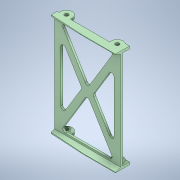
# Autodesk Inventor part: BodyStructure Plate
Saved by Autodesk Inventor 2022.2 (Build 262287000, 287)
## iProperties
Created: 2019-11-07
Part Number: BodyStructure Plate
Material: solidworks materials|ABS
Document SubType Name: Modeling
Designer: Jochen
Density: 1.02 g/cm^3
Appearance: 151,157,178
Sending System: SolidWorks 2017
Last Author: Felix
Last Saved: 2021-02-23
Author: Jochen
Autodesk Inventor part; units mm, degrees
ref_plane "YZ Plane" through (0, 0, 0) normal (1, 0, 0) x (0, 1, 0)
ref_plane "XZ Plane" through (0, 0, 0) normal (0, 1, 0) x (-1, 0, 0)
ref_plane "Work Plane1" through (0, 0, 30) normal (0, 0, 1) x (1, 0, 0)
sketch "Sketch1" plane through (0, 0, 30) normal (0, 0, 1) x (1, 0, 0)
  line L0 (-26, -40.5) -> (26, -40.5)
  line L1 (26, 40.5) -> (-26, 40.5)
  line L2 (26, 37) -> (26, 37)
  line L3 (0, -56.7) -> (0, 56.7) construction
  line L4 (-36.4, 0) -> (36.4, 0) construction
  line L5 (0, -2.5) -> (-21, -37)
  line L6 (-21, -27.3836) -> (-4.3317, 0)
  line L7 (-21, 27.3836) -> (-4.3317, 0)
  line L8 (0, 2.5) -> (-21, 37)
  line L9 (-26, 37) -> (-26, 37)
  line L10 (-21, 37) -> (21, 37)
  line L11 (-26, -37) -> (-26, -37)
  line L12 (21, -37) -> (-21, -37)
  line L13 (26, -37) -> (26, -37)
  line L14 (26, -40.5) -> (26, -37)
  line L15 (26, 37) -> (26, 40.5)
  line L16 (-26, 40.5) -> (-26, 37)
  line L17 (-26, -37) -> (-26, -40.5)
  line L18 (-26, -37) -> (-26, 37)
  line L19 (-21, -27.3836) -> (-21, 27.3836)
  line L20 (26, -37) -> (26, 37)
  line L21 (21, -27.3836) -> (21, 27.3836)
  line L22 (0, -2.5) -> (21, -37)
  line L23 (21, -27.3836) -> (4.3317, 0)
  line L24 (4.3317, 0) -> (21, 27.3836)
  line L25 (21, 37) -> (0, 2.5)
  point P0 (0, 0)
  point P1 (-5.9128, 0)
  dimension "d1" = 5
  dimension "d3" = 0
  dimension "d4" = 52
  dimension "d7" = 81
  dimension "d81" = 3.5
  dimension "d82" = 5
  dimension "d83" = 5
  dimension "d84" = 5
  constraints: 48 end point, 7 parallel, 6 horizontal, 5 collinear, 4 perpendicular, 4 point on line, 3 vertical, 1 coincident, 13 other
  measures "d1" distance between parallel lines of L6 L5
  measures "d3" distance of L11.start L11.end
  measures "d4" distance of L0.start L0.end
  measures "d7" distance between parallel lines of L1 L0
  measures "d81" distance of L11.end L0.start
  measures "d82" distance between parallel lines of L19 L18
  measures "d83" distance of L8.start L5.start
  measures "d84" distance of L5.end L11.start
extrude "Extrusion1" add sketch "Sketch1" along normal blind 13
fillet "Fillet1" radius 2 12 edges at (21, -37, 36.5) (0, -2.5, 36.5) (-21, -37, 36.5) (-4.3317, 0, 36.5) (-21, 37, 36.5) (21, 37, 36.5) (4.3317, 0, 36.5) (0, 2.5, 36.5) (21, -27.3836, 36.5) (-21, -27.3836, 36.5) (-21, 27.3836, 36.5) (21, 27.3836, 36.5)
sketch "Sketch3" plane through (0, 0, 0) normal (1, 0, 0) x (0, 1, 0)
  line L0 (0, -8.6) -> (0, 51.6) construction
  line L1 (-56.794, 0) -> (56.7157, 0) construction
  line L2 (-40.5, 43) -> (40.5, 43) construction
  line L3 (40.5, 43) -> (-40.5, 43) construction
  line L4 (21.2913, 43) -> (1.0399, 43) construction
  line L5 (-1.0399, 43) -> (1.0399, 43) construction
  line L6 (-1.0399, 43) -> (-21.2913, 43) construction
  line L7 (-1.0399, 30) -> (-21.2913, 30) construction
  line L8 (1.0399, 30) -> (-1.0399, 30) construction
  line L9 (21.2913, 30) -> (1.0399, 30) construction
  line L10 (40.5, 30) -> (-40.5, 30) construction
  line L11 (-40.5, 30) -> (40.5, 30) construction
  line L12 (40.5, 30) -> (40.5, 43) construction
  line L13 (40.5, 30) -> (40.5, 43) construction
  line L14 (37, 30) -> (37, 42.5) construction
  line L15 (37, 30) -> (37, 42.5) construction
  line L16 (-40.5, 30) -> (-40.5, 43) construction
  line L17 (-40.5, 30) -> (-40.5, 43) construction
  line L18 (-37, 30) -> (-37, 41) construction
  line L19 (-40.5, 30) -> (-40.5, 38.5)
  line L20 (-40.5, 43) -> (-40, 43)
  line L21 (-40, 43) -> (-38.5441, 39)
  line L22 (-38.5441, 39) -> (38.5441, 39)
  line L23 (40.5, 40.0648) -> (40.5, 30)
  line L24 (-40.25, 43) -> (-40.25, 30) construction
  line L25 (-20.2514, 30) -> (20.2514, 30) projected
  line L26 (-20.2514, 43) -> (20.2514, 43) projected
  line L27 (20.2514, 30) -> (21.2913, 30) projected
  line L28 (-21.2913, 30) -> (-20.2514, 30) projected
  line L29 (-20.2514, 43) -> (-21.2913, 43) projected
  line L30 (21.2913, 43) -> (20.2514, 43) projected
  line L31 (-40.5, 43) -> (-40.5, 38.5)
  line L32 (-38.5, 30) -> (-38.5, 37.5)
  line L33 (-38.5, 37.5) -> (-37, 37.5)
  line L34 (40.5, 30) -> (40.5, 43) projected
  line L35 (40.5, 40.0648) -> (40.5, 43)
  line L36 (40.5, 43) -> (40, 43)
  line L37 (40.5, 43) -> (-40.5, 43) projected
  line L38 (40, 43) -> (38.5441, 39)
  line L39 (38.5, 37.5) -> (38.5, 30)
  line L40 (37.0296, 37.5) -> (38.5, 37.5)
  line L41 (-37, 37.5) -> (37.0296, 37.5)
  line L42 (-40.5783, 30) -> (-38.5, 30)
  line L43 (40.5, 30) -> (-40.5, 30) projected
  point P0 (0, 0)
  point P1 (37, 41)
  point P2 (37, 41)
  point P3 (37, 41)
  point P4 (-37, 30)
  point P5 (37, 30)
  point P6 (-37, 30)
  point P7 (-40.5, 34.25)
  point P8 (-40, 43)
  dimension "d29" = 0.5
  dimension "d85" = 2
  dimension "d88" = 7.5
  dimension "d89" = 20
  dimension "d90" = 1.5
  constraints: 34 end point, 3 collinear, 2 horizontal, 2 midpoint, 2 perpendicular, 2 point on line, 1 parallel, 1 vertical, 7 other
  measures "d29" distance of L3.end L20.end
  measures "d85" distance between parallel lines of L32 L16
  measures "d88" distance of L32.start L32.end
  measures "d89" angle of L21 L16
  measures "d90" distance between parallel lines of L22 L41
extrude "Extrusion3" cut sketch "Sketch3" along normal through all both and the other way through all contours L19 L31 L20 L21 L22 L38 L36 L34 L23 L43 L39 L40 L41 L33 L32 L42 keep common part
sketch "Sketch11" plane through (0, 0, 0) normal (0, 1, 0) x (-1, 0, 0)
  line L0 (26, 43) -> (-26, 43) construction
  line L1 (1.3887, 42.8795) -> (26, 41.5273)
  line L2 (26, 41.5273) -> (26, 30)
  line L3 (26, 30) -> (26, 43) construction
  line L4 (6, 30) -> (26, 30)
  arc A0 (1.3887, 42.8795) -> (-3, 43) centre (-3, -37) ccw
  line L5 (-26, 30) -> (26, 30) construction
  line L6 (-26, 43) -> (-26, 39) projected
  line L7 (26, 41.5273) -> (72, 39) construction
  line L8 (-3, 43) -> (-26, 43)
  line L9 (-26, 43) -> (-26, 30)
  line L10 (-26, 30) -> (6, 30)
  line L11 (26, 30) -> (-26, 30) projected
  line L12 (26, 37.5) -> (21, 37.5) projected
  line L13 (21, 37.5) -> (21, 39) projected
  line L14 (21, 39) -> (26, 39) projected
  line L15 (26, 39) -> (26, 37.5) projected
  line L16 (4.6731, 37.5) -> (-4.6731, 37.5) projected
  line L17 (-4.6731, 37.5) -> (-4.6731, 39) projected
  line L18 (-4.6731, 39) -> (4.6731, 39) projected
  line L19 (4.6731, 39) -> (4.6731, 37.5) projected
  line L20 (-21, 37.5) -> (-26, 37.5) projected
  line L21 (-26, 37.5) -> (-26, 39) projected
  line L22 (-26, 39) -> (-21, 39) projected
  line L23 (-21, 39) -> (-21, 37.5) projected
  point P0 (0, 0)
  dimension "d91" = 80
  dimension "d93" = 98
  dimension "d94" = 4
  dimension "d95" = 23
  constraints: 14 end point, 3 point on line, 2 collinear, 2 point on circle, 2 tangent, 1 centre point, 1 vertical
  measures "d91" radius of A0
  measures "d93" horizontal distance of L7.end L0.end
  measures "d94" distance from line of L0 L7.end
  measures "d95" distance from line of L8.start L6
extrude "Extrusion11" cut sketch "Sketch11" along normal through all both and the other way through all contours L1 L2 L14 L13 L12 L4 L10 L9 L20 L23 L22 L6 L8 A0 | L2 L12 L13 L14 | L22 L23 L20 L9 | L16 L17 L18 L19 keep common part
sketch "Sketch12" plane through (0, 0, 0) normal (0, 1, 0) x (-1, 0, 0)
  circle A0 centre (-20, 35.5) radius 1.5
  circle A1 centre (-20, 35.5) radius 3
  circle A2 centre (20, 35.5) radius 1.5
  circle A3 centre (20, 35.5) radius 3
  line L0 (-26, 37.5) -> (-26, 30) construction
  line L1 (-20, 35.5) -> (20, 35.5) construction
  line L2 (26, 30) -> (26, 37.5) construction
  line L3 (25.5, 37) -> (26, 37)
  line L4 (26, 30) -> (26, 37)
  arc A4 (22.8284, 32) -> (24.5, 35.5) centre (20, 35.5) ccw
  arc A5 (15.5, 35.5) -> (22.8284, 32) centre (20, 35.5) ccw
  line L5 (15.5, 37) -> (-15.5, 37)
  arc A6 (-22.8284, 32) -> (-15.5, 35.5) centre (-20, 35.5) ccw
  line L6 (24.5, 35.5) -> (24.5, 36)
  arc A7 (25.5, 37) -> (24.5, 36) centre (25.5, 36) ccw
  arc A8 (22.8284, 32) -> (22.8284, 32) centre (19.5074, 36.1096) ccw
  line L7 (-26, 32) -> (-22.8284, 32)
  line L8 (-26, 43) -> (-26, 32)
  line L9 (-26, 43) -> (26, 43)
  line L10 (26, 37) -> (26, 43)
  line L11 (26, 39) -> (-26, 39) projected
  line L12 (-22.8284, 39) -> (22.9247, 39)
  arc A9 (-24.5, 35.5) -> (-22.8284, 32) centre (-20, 35.5) ccw
  line L13 (15.5, 35.5) -> (15.5, 37)
  line L14 (24.5, 36) -> (24.5, 37.5)
  line L15 (24.5, 37.5) -> (22.2361, 37.5)
  line L16 (-24.5, 37) -> (-24.5, 35.5)
  line L17 (-15.5, 37) -> (-15.5, 35.5)
  line L18 (-26, 37.5) -> (26, 37.5) projected
  line L19 (-22.2361, 37.5) -> (-24.5, 37.5)
  line L20 (-24.5, 37) -> (-24.5, 37.5)
  line L21 (-17.7639, 37.5) -> (-15.5, 37.5)
  line L22 (-19.1496, 37.5) -> (-1.7084, 37.5) projected
  line L23 (-15.5, 37) -> (-15.5, 36.8517)
  line L24 (-15.5, 37) -> (-15.5, 37.5)
  line L25 (15.5, 37) -> (15.5, 37.5)
  line L26 (17.4412, 37.5) -> (-17.4412, 37.5) projected
  line L27 (15.5, 37.5) -> (17.7639, 37.5)
  line L28 (1.7084, 37.5) -> (19.1496, 37.5) projected
  point P0 (0, 0)
  point P1 (24.5, 37)
  point P2 (-24.4142, 32)
  point P3 (22.8284, 32)
  point P4 (17.4019, 37)
  point P5 (-17.4019, 37)
  point P6 (-22.5981, 37)
  dimension "d98" = 3
  dimension "d99" = 6
  dimension "d100" = 6
  dimension "d101" = 6
  dimension "d102" = 7.5
  dimension "d110" = 4.5
  dimension "d111" = 1
  dimension "d113" = 6
  dimension "d114" = 11
  constraints: 44 end point, 19 point on circle, 12 point on line, 10 centre point, 7 tangent, 6 coincident, 6 vertical, 5 equal radius, 4 perpendicular, 3 horizontal, 2 collinear, 1 midpoint, 5 other
  measures "d98" diameter of A0
  measures "d99" diameter of A1
  measures "d100" distance from line of L1.start L0
  measures "d101" distance from line of A2.centre L2
  measures "d102" vertical distance of L8.start A0.centre
  measures "d110" radius of A4
  measures "d111" radius of A7
  measures "d113" distance between parallel lines of L9 L5
  measures "d114" distance between parallel lines of L9 L7
extrude "Extrusion12" cut sketch "Sketch12" along normal through all both and the other way through all contours A0 | A2
extrude "Extrusion13" cut sketch "Sketch12" along normal through all both and the other way through all contours A0 | A1 L18 | A1 L18 L24 L17 A6 A9 L16 L20 | L18 A1 | A1 L18 L8 L11 A8 | L20 L16 A9 L7 L8 L18 | L18 A8 L5 L24 | L8 L9 L10 L11 A8 | A8 L18 L25 L5 | A8 L11 L18 L15 A3 | L25 L18 A3 L15 L14 L6 A4 A5 L13 | A8 L11 | L10 L18 A8 L11 | L14 L18 A8 A7 | A8 L18 L10 L3 A7 | L18 A3 | A3 L18 | A2 keep common part
extrude "Extrusion14" add sketch "Sketch12" along normal blind 1 from surface at -38.5 contours A1 L18 | A1 L18 L24 L17 A6 A9 L16 L20 | L18 A1 | L25 L18 A3 L15 L14 L6 A4 A5 L13 | L18 A3 | A3 L18
extrude "Extrusion15" add sketch "Sketch12" against normal blind 1 from surface at 38.5 contours A1 L18 | A1 L18 L24 L17 A6 A9 L16 L20 | L18 A1 | L25 L18 A3 L15 L14 L6 A4 A5 L13 | L18 A3 | A3 L18
chamfer "Chamfer2" distance 1 distance2 2 1 edges at (20, -37.5, 31) measured on face at (20, -38, 31)
chamfer "Chamfer3" distance 1 distance2 2 1 edges at (20, 37.5, 31) measured on face at (20, 38, 31)
chamfer "Chamfer4" distance 2 distance2 1 2 edges at (-20, 37.5, 31) (-24.5, 37.5, 36.5) measured on face at (-20, 37.5, 31.5) measured on face at (-24, 37.5, 36.5)
chamfer "Chamfer5" distance 2 distance2 1 3 edges at (-20, -37.5, 31) (-15.5, -37.5, 36.5) (-24.5, -37.5, 36.5) measured on face at (-24, -37.5, 36.5) measured on face at (-16, -37.5, 36.5) measured on face at (-20, -37.5, 31.5)
body "Solid1"
body "Solid2"
